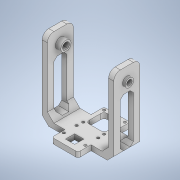
# Autodesk Inventor part: HoseMount
Saved by Autodesk Inventor 2020 (Build 240168000, 168)
## iProperties
Created: 2019-04-27
Part Number: HoseMount
Material: Generic
Document SubType Name: Modeling
Designer: Connor
Density: 1 g/cm^3
Appearance: Default
Author: Connor
Autodesk Inventor part; units mm, degrees
ref_plane "YZ Plane" through (0, 0, 0) normal (1, 0, 0) x (0, 1, 0)
ref_plane "XZ Plane" through (0, 0, 0) normal (0, 1, 0) x (-1, 0, 0)
ref_plane "XY Plane" through (0, 0, 0) normal (0, 0, 1) x (1, 0, 0)
sketch "Sketch1" plane through (0, 0, 0) normal (0, 0, 1) x (1, 0, 0)
  line L0 (0, 0) -> (69.85, 0)
  line L1 (69.85, 0) -> (69.85, 76.2)
  line L2 (0, 76.2) -> (0, 0)
  line L3 (64.77, 76.2) -> (64.77, 5.08)
  line L4 (64.77, 5.08) -> (5.08, 5.08)
  line L5 (5.08, 5.08) -> (5.08, 76.2)
  line L6 (69.85, 76.2) -> (64.77, 76.2)
  line L7 (5.08, 76.2) -> (0, 76.2)
  dimension "d0" = 69.85
  dimension "d1" = 5.08
  dimension "d2" = 5.08
  dimension "d3" = 76.2
  constraints: 16 end point, 4 parallel, 2 collinear, 1 horizontal, 1 perpendicular
  measures "d0" distance between parallel lines of L1 L2
  measures "d1" distance of L5.end L2.start
  measures "d2" distance between parallel lines of L0 L4
  measures "d3" distance of L0.end L1.end
extrude "Extrusion1" add sketch "Sketch1" along normal blind 25.4
sketch "Sketch2" plane through (0, 0, 0) normal (0, -1, 0) x (1, 0, 0)
  line L0 (22.225, 38.1) -> (47.625, 38.1)
  line L1 (47.625, 38.1) -> (47.625, -12.7)
  line L2 (47.625, -12.7) -> (22.225, -12.7)
  line L3 (22.225, -12.7) -> (22.225, 38.1)
  line L4 (0, 25.4) -> (69.85, 25.4) construction
  line L5 (0, 25.4) -> (22.225, 38.1) construction
  line L6 (0, 0) -> (69.85, 0) construction
  line L7 (0, 0) -> (22.225, -12.7) construction
  line L8 (47.625, 38.1) -> (69.85, 25.4) construction
  line L9 (47.625, -12.7) -> (69.85, 0) construction
  dimension "d6" = 50.8
  dimension "d7" = 25.4
  constraints: 16 end point, 2 equal length, 2 parallel, 1 horizontal, 1 perpendicular
  measures "d6" distance of L0.end L1.end
  measures "d7" distance between parallel lines of L1 L3
extrude "Extrusion2" add sketch "Sketch2" against normal up to surface (5.08 mm away)
sketch "Sketch3" plane through (69.85, 0, 0) normal (0, -1, 0) x (1, 0, 0)
  line L0 (-22.225, 38.1) -> (-47.625, 38.1) construction
  line L1 (-47.425, 38.1) -> (-22.425, 38.1) construction
  line L2 (-22.425, 38.1) -> (-22.425, 14.238) construction
  line L3 (-22.425, 14.238) -> (-47.425, 14.238) construction
  line L4 (-47.425, 14.238) -> (-47.425, 38.1) construction
  line L5 (-5.08, 25.4) -> (-22.225, 25.4) construction
  line L6 (-22.225, 25.4) -> (-22.425, 25.4) construction
  line L7 (-69.85, 25.4) -> (-47.625, 25.4) construction
  line L8 (-47.625, 25.4) -> (-47.425, 25.4) construction
  circle A0 centre (-45.425, 16.238) radius 1.25
  circle A1 centre (-24.425, 16.238) radius 1.25
  circle A2 centre (-45.425, 28.738) radius 1.25
  circle A3 centre (-24.425, 28.738) radius 1.25
  line L9 (-39.425, 33.138) -> (-30.425, 33.138)
  line L10 (-30.425, 33.138) -> (-30.425, 24.138)
  line L11 (-30.425, 24.138) -> (-39.425, 24.138)
  line L12 (-39.425, 24.138) -> (-39.425, 33.138)
  line L13 (-39.425, 33.138) -> (-30.425, 24.138) construction
  line L14 (-39.425, 24.138) -> (-30.425, 33.138) construction
  point P0 (-69.85, 0)
  point P1 (-34.925, 28.638)
  dimension "d10" = 23.862
  dimension "d11" = 25
  dimension "d12" = 2.5
  dimension "d13" = 2
  dimension "d14" = 2
  dimension "d15" = 2
  dimension "d16" = 14.5
  dimension "d17" = 9
  dimension "d18" = 9.462
  dimension "d19" = 12.5
  constraints: 24 end point, 4 centre point, 4 parallel, 4 perpendicular, 4 point on line, 3 equal radius, 2 equal length, 2 horizontal, 2 horizontal alignment, 2 vertical alignment, 1 midpoint
  measures "d10" distance of L1.end L2.end
  measures "d11" distance between parallel lines of L2 L4
  measures "d12" diameter of A0
  measures "d13" distance from line of L2 A1.centre
  measures "d14" distance from line of L3 A1.centre
  measures "d15" distance from line of L4 A0.centre
  measures "d16" distance from line of L3 A3.centre
  measures "d17" distance of L9.start L9.end
  measures "d18" distance from line of L1 point (-34.925, 28.638)
  measures "d19" distance from line of L2 point (-34.925, 28.638)
extrude "Extrusion3" cut sketch "Sketch3" against normal up to surface (5.08 mm away)
sketch "Sketch4" plane through (0, 0, 0) normal (0, -1, 0) x (1, 0, 0)
  line L0 (22.225, 0) -> (22.225, -12.7) construction
  line L1 (22.225, -12.7) -> (47.625, -12.7) construction
  line L2 (47.625, -12.7) -> (47.625, 12.7) construction
  line L3 (47.625, 12.7) -> (22.225, 12.7) construction
  line L4 (22.225, 12.7) -> (22.225, -12.7) construction
  line L5 (47.625, -12.7) -> (47.625, 0) construction
  line L6 (22.225, 12.7) -> (47.625, -12.7) construction
  line L7 (47.625, 12.7) -> (22.225, -12.7) construction
  line L8 (26.035, 8.89) -> (43.815, 8.89)
  line L9 (43.815, 8.89) -> (43.815, -8.89)
  line L10 (43.815, -8.89) -> (26.035, -8.89)
  line L11 (26.035, -8.89) -> (26.035, 8.89)
  circle A0 centre (24.765, 10.16) radius 1.25
  circle A1 centre (45.085, 10.16) radius 1.25
  circle A2 centre (45.085, -10.16) radius 1.25
  circle A3 centre (24.765, -10.16) radius 1.25
  point P0 (0, 0)
  dimension "d22" = 2.5
  dimension "d23" = 20.32
  dimension "d24" = 17.78
  constraints: 20 end point, 7 point on line, 4 centre point, 4 parallel, 4 perpendicular, 3 equal radius, 2 horizontal, 2 vertical alignment, 1 collinear, 1 horizontal alignment
  measures "d22" diameter of A0
  measures "d23" distance of A1.centre A0.centre
  measures "d24" distance of L8.start L8.end
extrude "Extrusion4" cut sketch "Sketch4" against normal up to surface (5.08 mm away)
sketch "Sketch5" plane through (0, 0, 0) normal (-1, 0, 0) x (0, 0, 1)
  line L0 (0, 76.2) -> (25.4, 76.2) construction
  line L1 (0, 76.2) -> (0, 5.08) construction
  line L2 (25.4, 76.2) -> (0, 76.2) construction
  line L3 (0, 76.2) -> (0, 50.8) construction
  line L4 (0, 50.8) -> (25.4, 50.8) construction
  line L5 (25.4, 50.8) -> (25.4, 76.2) construction
  line L6 (25.4, 76.2) -> (0, 50.8) construction
  line L7 (25.4, 50.8) -> (0, 76.2) construction
  arc A0 (14.4861, 60.875) -> (10.9139, 60.875) centre (12.7, 63.5) ccw construction
  line L8 (14.4861, 60.875) -> (10.9139, 60.875) construction
  line L9 (10.8534, 60.675) -> (14.5466, 60.675)
  arc A1 (14.5466, 60.675) -> (10.8534, 60.675) centre (12.7, 63.5) ccw
  point P0 (0, 0)
  dimension "d27" = 25.4
  dimension "d28" = 6.35
  dimension "d29" = 5.8
  dimension "d54" = 0.2
  constraints: 16 end point, 4 point on circle, 2 centre point, 2 horizontal, 2 parallel, 1 midpoint, 1 perpendicular, 1 point on line, 1 other
  measures "d27" distance between parallel lines of L0 L4
  measures "d28" diameter of A0
  measures "d54" radial gap between concentric circles of A0 A1
extrude "Extrusion5" cut sketch "Sketch5" against normal up to surface (5.08 mm away)
sketch "Sketch6" plane through (69.85, 0, 0) normal (1, 0, 0) x (0, 0, -1)
  line L0 (-25.4, 76.2) -> (-25.4, 0) construction
  line L1 (-25.4, 76.2) -> (0, 50.8) construction
  line L2 (0, 76.2) -> (0, 0) construction
  line L3 (0, 76.2) -> (-25.4, 76.2) construction
  line L4 (0, 76.2) -> (-25.4, 50.8) construction
  line L5 (-25.4, 0) -> (-25.4, 76.2) construction
  line L6 (-25.4, 50.8) -> (0, 50.8) construction
  line L7 (-25.4, 5.08) -> (-25.4, 76.2) projected
  circle A0 centre (-12.7, 63.5) radius 2.6035
  dimension "d52" = 25.4
  dimension "d53" = 5.207
  constraints: 6 end point, 2 perpendicular, 2 point on line, 1 centre point, 1 midpoint
  measures "d52" distance between parallel lines of L3 L6
  measures "d53" diameter of A0
extrude "Extrusion6" cut sketch "Sketch6" against normal up to surface (5.08 mm away)
fillet "Fillet1" radius 2 4 edges at (47.625, 2.54, 38.1) (22.225, 2.54, 38.1) (22.225, 2.54, -12.7) (47.625, 2.54, -12.7)
fillet "Fillet2" radius 6.35 4 edges at (67.31, 76.2, 25.4) (67.31, 76.2, 0) (2.54, 76.2, 25.4) (2.54, 76.2, 0)
chamfer "Chamfer1" distance 6.35 angle 45 4 edges at (0, 0, 12.7) (5.08, 5.08, 12.7) (69.85, 0, 12.7) (64.77, 5.08, 12.7)
sketch "Sketch7" plane through (0, 76.2, 6.35) normal (-1, 0, 0) x (0, 0, 1)
  line L0 (12.7, -22.225) -> (0, -22.225)
  line L1 (0, -22.225) -> (0, -69.85)
  line L2 (0, -69.85) -> (12.7, -69.85)
  line L3 (12.7, -69.85) -> (12.7, -22.225)
  line L4 (-6.35, -6.35) -> (-6.35, -69.85) projected
  line L5 (19.05, -69.85) -> (-6.35, -69.85) projected
  line L6 (19.05, -6.35) -> (19.05, -69.85) projected
  arc A0 (8.975, -10.9139) -> (8.975, -14.4861) centre (6.35, -12.7) ccw projected
  point P0 (-6.35, -76.2)
  dimension "d42" = 6.35
  dimension "d43" = 0
  dimension "d44" = 6.35
  dimension "d46" = 6.35
  constraints: 8 end point, 2 parallel, 1 horizontal, 1 perpendicular
  measures "d42" distance between parallel lines of L4 L1
  measures "d43" distance between parallel lines of L5 L2
  measures "d44" distance between parallel lines of L3 L6
  measures "d46" distance edge to line of A0 L0
extrude "Extrusion7" cut sketch "Sketch7" against normal through all
chamfer "Chamfer2" distance 3.175 angle 45 8 edges at (64.77, 6.35, 19.05) (64.77, 6.35, 6.35) (67.31, 53.975, 6.35) (67.31, 53.975, 19.05) (5.08, 6.35, 6.35) (5.08, 6.35, 19.05) (2.54, 53.975, 19.05) (2.54, 53.975, 6.35)
fillet "Fillet3" radius 3.175 4 edges at (26.035, 2.54, 8.89) (26.035, 2.54, -8.89) (43.815, 2.54, -8.89) (43.815, 2.54, 8.89)
sketch "Sketch8" plane through (0, 76.2, 6.35) normal (-1, 0, 0) x (0, 0, 1)
  arc A0 (8.1966, -15.525) -> (4.5034, -15.525) centre (6.35, -12.7) ccw projected
  line L0 (8.1966, -15.525) -> (4.5034, -15.525) projected
  arc A1 (8.6238, -17.125) -> (4.0762, -17.125) centre (6.35, -12.7) ccw
  line L1 (8.6238, -17.125) -> (4.0762, -17.125)
  point P0 (-6.35, -76.2)
  dimension "d56" = 1.6
  constraints: 2 end point, 2 point on circle, 1 centre point, 1 other
  measures "d56" radial gap between concentric circles of A0 A1
extrude "Extrusion8" add sketch "Sketch8" along normal blind 4.525
sketch "Sketch9" plane through (5.08, 76.2, 19.05) normal (1, 0, 0) x (0, 0, -1)
  line L0 (8.1966, -15.525) -> (4.5034, -15.525) projected
  arc A0 (8.1966, -15.525) -> (4.5034, -15.525) centre (6.35, -12.7) ccw projected
  line L1 (4.0762, -17.125) -> (8.6238, -17.125)
  arc A1 (8.6238, -17.125) -> (4.0762, -17.125) centre (6.35, -12.7) ccw
  point P0 (19.05, -76.2)
  dimension "d59" = 1.6
  constraints: 2 end point, 2 point on circle, 1 centre point, 1 other
  measures "d59" radial gap between concentric circles of A0 A1
extrude "Extrusion9" add sketch "Sketch9" along normal blind 5.4
sketch "Sketch10" plane through (69.85, 76.2, 19.05) normal (1, 0, 0) x (0, 0, -1)
  circle A0 centre (6.35, -12.7) radius 2.6035 projected
  circle A1 centre (6.35, -12.7) radius 4.2035
  point P0 (19.05, -76.2)
  dimension "d62" = 1.6
  constraints: 1 centre point
  measures "d62" radial gap between concentric circles of A0 A1
extrude "Extrusion10" add sketch "Sketch10" along normal blind 2.54
body "Solid1"
